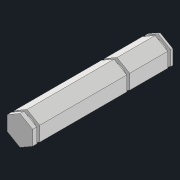
# Autodesk Inventor part: Performance Axle
Saved by Autodesk Inventor 2022 (Build 260153000, 153)
## iProperties
Created: 2022-09-07
Part Number: Performance Axle
Material: Generic
Document SubType Name: Modeling
Designer: robpl
Density: 1 g/cm^3
Appearance: Default
Author: robpl
Autodesk Inventor part; units mm, degrees
ref_plane "YZ Plane" through (0, 0, 0) normal (1, 0, 0) x (0, 1, 0)
ref_plane "XZ Plane" through (0, 0, 0) normal (0, 1, 0) x (-1, 0, 0)
ref_plane "XY Plane" through (0, 0, 0) normal (0, 0, 1) x (1, 0, 0)
sketch "Sketch1" plane through (0, 0, 0) normal (0, 0, 1) x (1, 0, 0)
  line L0 (6.35, 3.6662) -> (6.35, -3.6662)
  line L1 (6.35, -3.6662) -> (0, -7.3323)
  line L2 (0, -7.3323) -> (-6.35, -3.6662)
  line L3 (-6.35, -3.6662) -> (-6.35, 3.6662)
  line L4 (-6.35, 3.6662) -> (0, 7.3323)
  line L5 (0, 7.3323) -> (6.35, 3.6662)
  point P0 (0, 0)
  point P1 (0, 0)
  dimension "d0" = 12.7
  constraints: 12 end point, 1 coincident, 1 vertical, 13 other
  measures "d0" distance between parallel lines of L3 L0
extrude "Extrusion1" add sketch "Sketch1" along normal blind 71
sketch "Sketch2" plane through (0, 0, 0) normal (0, 1, 0) x (-1, 0, 0)
  line L0 (15, 67.5) -> (5, 67.5)
  line L1 (5, 67.5) -> (5, 69)
  line L2 (5, 69) -> (15, 69)
  line L3 (15, 69) -> (15, 67.5)
  line L4 (15, 22.5) -> (5, 22.5)
  line L5 (5, 22.5) -> (5, 24)
  line L6 (5, 24) -> (15, 24)
  line L7 (15, 24) -> (15, 22.5)
  line L8 (15, 1.5) -> (5, 1.5)
  line L9 (5, 1.5) -> (5, 3)
  line L10 (5, 3) -> (15, 3)
  line L11 (15, 3) -> (15, 1.5)
  line L12 (0, 71) -> (6.35, 71) projected
  line L13 (0, 0) -> (0, 71) projected
  line L14 (0, -14) -> (0, 84) projected
  dimension "d3" = 2
  dimension "d4" = 1.5
  dimension "d5" = 47
  dimension "d6" = 68
  dimension "d7" = 10
  dimension "d8" = 5
  constraints: 24 end point, 6 parallel, 3 equal length, 3 horizontal, 3 perpendicular, 3 point on line
  measures "d3" distance between parallel lines of L12 L2
  measures "d4" distance of L2.end L0.start
  measures "d5" distance between parallel lines of L12 L6
  measures "d6" distance between parallel lines of L10 L12
  measures "d7" distance of L8.start L8.end
  measures "d8" distance from line of L13 L9.end
revolve "Revolution1" cut sketch "Sketch2" angle 360 about axis through (0, 0, -10) along (0, 0, 1)
body "Solid1"
